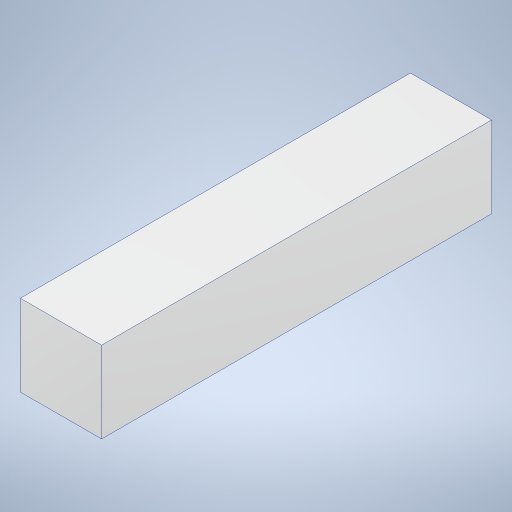
# Autodesk Inventor part: rapoukLegSupportv1
Saved by Autodesk Inventor 2024 (Build 280153000, 153)
## iProperties
Created: 2023-06-23
Part Number: rapoukLegSupportv1
Material: Aluminum 6061
Document SubType Name: Modeling
Designer: Roman
Density: 2.7 g/cm^3
Appearance: Aluminum - Flat
Description: Podpůrný sloupek
Mass: 0.72 g
Surface Area: 5.88 cm^2
Volume: 0.72 cm^3
Polotovar: KR...
Author: Roman
Autodesk Inventor part; units mm, degrees
ref_plane "YZ Plane" through (0, 0, 0) normal (1, 0, 0) x (0, 1, 0)
ref_plane "XZ Plane" through (0, 0, 0) normal (0, 1, 0) x (-1, 0, 0)
ref_plane "XY Plane" through (0, 0, 0) normal (0, 0, 1) x (1, 0, 0)
sketch "Sketch1" plane through (0, 0, 0) normal (0, 1, 0) x (-1, 0, 0)
  line L0 (-2.5, 12) -> (2.5, 12)
  line L1 (2.5, 12) -> (2.5, -12)
  line L2 (2.5, -12) -> (-2.5, -12)
  line L3 (-2.5, -12) -> (-2.5, 12)
  line L4 (-2.5, 12) -> (2.5, -12) construction
  line L5 (2.5, 12) -> (-2.5, -12) construction
  point P0 (0, 0)
  dimension "d0" = 5
  dimension "d1" = 24
  constraints: 12 end point, 2 midpoint, 2 parallel, 1 horizontal, 1 perpendicular
  measures "d0" distance of L1.end L2.end
  measures "d1" distance of L0.end L1.end
extrude "Extrusion1" add sketch "Sketch1" along normal blind 5
body "Solid1"
